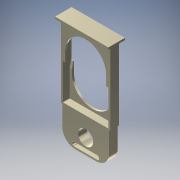
# Autodesk Inventor part: Cup_Dispenser_Slider
Saved by Autodesk Inventor 2016 (Build 200138000, 138)
## iProperties
Created: 2015-07-03
Part Number: Cup_Dispenser_Slider
Material: Generic
Document SubType Name: Modeling
Designer: bastli
Density: 1 g/cm^3
Appearance: Nickel
Author: bastli
Autodesk Inventor part; units mm, degrees
ref_plane "YZ Plane" through (0, 0, 0) normal (1, 0, 0) x (0, 1, 0)
ref_plane "XZ Plane" through (0, 0, 0) normal (0, 1, 0) x (-1, 0, 0)
ref_plane "XY Plane" through (0, 0, 0) normal (0, 0, 1) x (1, 0, 0)
sketch "Sketch13" plane through (0, 0, 0) normal (0, 1, 0) x (-1, 0, 0)
  circle A0 centre (0, 0) radius 35 construction
  circle A1 centre (0, 0) radius 31.375 construction
  line L0 (0, 60.7625) -> (0, -56.1294) construction
  line L1 (45.182, 0) -> (-48.0239, 0) construction
  circle A2 centre (0, 35) radius 35 construction
  circle A3 centre (0, 35) radius 31.375 construction
  line L2 (31.375, 35) -> (31.375, 19.4884)
  line L3 (35, 19.4884) -> (35, 70)
  line L4 (35, 70) -> (0, 70)
  line L5 (31.375, 19.4884) -> (35, 19.4884)
  arc A4 (31.375, 35) -> (0, 66.375) centre (0, 35) ccw
  line L6 (0, 70) -> (0, 66.375) construction
  line L7 (0, 31.375) -> (0, 3.625) construction
  line L8 (0, 17.5) -> (45.182, 17.5) construction
  line L9 (-31.375, 35) -> (-31.375, 19.4884)
  line L10 (-35, 19.4884) -> (-35, 70)
  line L11 (-35, 70) -> (0, 70)
  line L12 (-31.375, 19.4884) -> (-35, 19.4884)
  arc A5 (0, 66.375) -> (-31.375, 35) centre (0, 35) ccw
  line L13 (31.375, 0) -> (31.375, 15.5116)
  line L14 (35, 15.5116) -> (35, -35)
  line L15 (35, -35) -> (0, -35)
  line L16 (31.375, 15.5116) -> (35, 15.5116)
  arc A6 (0, -31.375) -> (31.375, 0) centre (0, 0) ccw
  line L17 (-35, 15.5116) -> (-35, -35)
  line L18 (-35, -35) -> (0, -35)
  line L19 (-31.375, 15.5116) -> (-35, 15.5116)
  line L20 (-31.375, 0) -> (-31.375, 15.5116)
  arc A7 (-31.375, 0) -> (0, -31.375) centre (0, 0) ccw
  line L21 (35, 70) -> (35, -35)
  line L22 (-35, -35) -> (-35, 70)
  line L23 (-38, 73) -> (38, 73)
  line L24 (38, 73) -> (38, -38)
  line L25 (38, -38) -> (-38, -38)
  line L26 (-38, -38) -> (-38, 73)
  line L27 (-38, 73) -> (38, -38) construction
  line L28 (38, 73) -> (-38, -38) construction
  dimension "d49" = 70
  dimension "d50" = 62.75
  dimension "d51" = 70
  dimension "d53" = 62.75
  dimension "d54" = 76
  dimension "d55" = 111
  constraints: 58 end point, 15 symmetric about line, 13 point on circle, 6 centre point, 6 point on line, 4 coincident, 4 parallel, 4 perpendicular, 3 horizontal, 3 midpoint, 3 tangent, 2 vertical alignment, 1 collinear, 1 vertical, 7 other
  measures "d51" diameter of A2
  measures "d53" diameter of A3
  measures "d54" distance of L24.end L25.end
  measures "d55" distance of L23.end L24.end
extrude "Extrusion11" add sketch "Sketch13" against normal blind 3 contours L14 L15 L18 L17 L19 L20 A7 A6 L13 L16 | L23 L24 L25 L26
extrude "Extrusion12" add sketch "Sketch13" against normal blind 10.5
sketch "Sketch14" plane through (0, -10.5, 0) normal (0, -1, 0) x (1, 0, 0)
  arc A0 (31.375, 35) -> (0, 66.375) centre (0, 35) ccw projected
  line L0 (31.375, 35) -> (31.375, 19.4884) projected
  line L1 (31.375, 19.4884) -> (35, 19.4884) projected
  arc A1 (0, 66.375) -> (-31.375, 35) centre (0, 35) ccw projected
  line L2 (-31.375, 35) -> (-31.375, 19.4884) projected
  line L3 (-31.375, 19.4884) -> (-35, 19.4884) projected
  line L4 (-35, 70) -> (35, 70) projected
  line L5 (35, 70) -> (35, -35) projected
  line L6 (-35, -35) -> (-35, 70) projected
  line L7 (35, 70) -> (35, -35) projected
  line L8 (35, -35) -> (-35, -35) projected
  line L9 (-35, -35) -> (-35, 70) projected
  line L10 (-35, 70) -> (35, 70) projected
  line L11 (38, 73) -> (-38, 73) projected
  line L12 (-38, 73) -> (-38, -38) projected
  line L13 (-38, -38) -> (38, -38) projected
  line L14 (38, -38) -> (38, 73) projected
  point P0 (0, 0)
extrude "Extrusion13" add sketch "Sketch14" along normal blind 3 contours A0 A1 L2 L3 L6 L4 L5 L1 L0 | L14 L13 L12 L11
chamfer "Chamfer3" distance 2 angle 45 2 edges at (-38, -6.75, -38) (38, -6.75, -38)
chamfer "Chamfer4" distance 10 distance2 2 1 edges at (33.1875, -3, 15.5116) measured on face at (33.1875, -3, 15.0116)
chamfer "Chamfer5" distance 10 distance2 2 1 edges at (-33.1875, -3, 15.5116) measured on face at (-33.1875, -3, 15.0116)
chamfer "Chamfer6" distance 2 distance2 10 1 edges at (-33.1875, -10.5, 19.4884) measured on face at (-33.1875, -11, 19.4884)
chamfer "Chamfer7" distance 2 distance2 10 1 edges at (33.1875, -10.5, 19.4884) measured on face at (33.1875, -11, 19.4884)
sketch "Sketch18" plane through (-35, 0, 70) normal (1, 0, 0) x (0, 0, -1)
  line L0 (38, -10.5) -> (35, -7.5)
  line L1 (35, -7.5) -> (32, -10.5)
  line L2 (40.5116, -10.5) -> (0, -10.5) projected
  line L3 (35, -10.5) -> (35, -13.5) construction
  line L4 (35, -10.5) -> (35, -7.5) construction
  point P0 (70, 0)
  dimension "d85" = 45
  dimension "d86" = 3
  constraints: 6 end point, 3 point on line, 1 perpendicular, 1 vertical
  measures "d85" angle of L2 L0
  measures "d86" distance from line of L2 L0.end
extrude "Extrusion17" add sketch "Sketch18" along normal up to surface (3.625 mm away)
mirror "Mirror4" about plane through (0, 0, 0) normal (1, 0, 0) of "Extrusion17"
sketch "Sketch15" plane through (-38, 0, 73) normal (0, 0, 1) x (1, 0, 0)
  line L0 (76, 0) -> (0, 0) projected
  line L1 (0, 0) -> (0, -13.5) projected
  line L2 (76, -13.5) -> (0, -13.5) projected
  line L3 (76, 0) -> (76, -13.5) projected
  point P0 (38, 0)
extrude "Extrusion14" add sketch "Sketch15" along normal blind 3
sketch "Sketch16" plane through (-38, 0, 76) normal (0, 0, 1) x (1, 0, 0)
  line L0 (76, 0) -> (0, 0) projected
  line L1 (0, 0) -> (0, -13.5) projected
  line L2 (0, -13.5) -> (76, -13.5) projected
  line L3 (76, -13.5) -> (76, 0) projected
  line L4 (76, 0) -> (76, -13.5) projected
  line L5 (76, -13.5) -> (0, -13.5) projected
  line L6 (0, -13.5) -> (0, 0) projected
  line L7 (0, 0) -> (76, 0) projected
  line L8 (-3, -19.5) -> (79, -19.5) projected
  line L9 (79, -19.5) -> (79, 6) projected
  line L10 (-3, 6) -> (79, 6) projected
  line L11 (-3, -19.5) -> (-3, 6) projected
  point P0 (38, 0)
extrude "Extrusion15" add sketch "Sketch16" along normal blind 3 contours L3 L2 L1 L0 | L11 L10 L9 L8
sketch "Sketch21" plane through (36, -13.5, -38) normal (0, 0, -1) x (-1, 0, 0)
  line L0 (0, 0) -> (0, 13.5) projected
  line L1 (72, 0) -> (0, 0) projected
  line L2 (72, 13.5) -> (72, 0) projected
  line L3 (72, 13.5) -> (0, 13.5) projected
  point P0 (36, 13.5)
extrude "Extrusion20" add sketch "Sketch21" along normal blind 50
sketch "Sketch22" plane through (0, -13.5, 0) normal (0, -1, 0) x (1, 0, 0)
  line L0 (36, -88) -> (-36, -88) projected
  line L1 (0, -88) -> (0, -22.6471) construction
  line L2 (-17.5, -82) -> (17.5, -82) construction
  line L3 (-17.5, -85) -> (17.5, -85)
  line L4 (17.5, -79) -> (-17.5, -79)
  arc A0 (-17.5, -79) -> (-17.5, -85) centre (-17.5, -82) ccw
  arc A1 (17.5, -85) -> (17.5, -79) centre (17.5, -82) ccw
  line L5 (-36, -38) -> (-36, -88) projected
  line L6 (36, -38) -> (36, -88) projected
  line L7 (-16, -88) -> (16, -88)
  line L8 (36, -68) -> (36, -38)
  line L9 (-38, -36) -> (-36, -38) projected
  line L10 (-36, -38) -> (-36, -68)
  arc A2 (16, -88) -> (36, -68) centre (16, -68) ccw
  arc A3 (-36, -68) -> (-16, -88) centre (-16, -68) ccw
  line L11 (-36, -68) -> (-36, -88)
  line L12 (-36, -88) -> (-16, -88)
  line L13 (-36, -88) -> (36, -88) projected
  line L14 (16, -88) -> (36, -88)
  line L15 (36, -88) -> (36, -68)
  circle A4 centre (0, -64.5) radius 11.5 projected
  point P0 (0, 0)
  point P1 (0, -82)
  dimension "d97" = 35
  dimension "d98" = 3
  dimension "d99" = 3
  dimension "d100" = 20
  constraints: 24 end point, 12 tangent, 8 point on circle, 6 point on line, 5 collinear, 4 centre point, 2 midpoint, 2 perpendicular, 1 equal radius, 1 parallel, 1 vertical
  measures "d97" distance of L2.end L2.start
  measures "d98" distance between parallel lines of L3 L2
  measures "d99" distance between parallel lines of L3 L0
  measures "d100" radius of A2
extrude "Extrusion21" cut sketch "Sketch22" against normal up to surface (13.5 mm away)
chamfer "Chamfer8" distance 1 angle 45 4 edges at (20.5, 0, -82) (0, 0, -79) (-20.5, 0, -82) (0, 0, -85)
thicken "Thicken1" operation add thickness 0.1 both sides no extend neighbours yes toward (0, 0, 1) faces at (12.6667, -17.5, 76) (-0.4621, -13.5, -41.0279) (-27.3942, 0, -55.0519) (-38, -9, 38.6667) (38, -9, 1.3333) (36, -4.5, -58) (32.5248, -4.5, -79.2664) (5.3333, -4.5, -88) (5.8333, -9.3333, -79) (-17.9812, -5.1667, -79.0388) (-33.3205, -4.5, -78) (20.4976, -5.1667, -81.8792) (-5.8333, -9.3333, -85) (-36, -9, -58) (-37.3333, -4.5, -36.6667) (37.3333, -9, -36.6667)
equation "\"printer_offset\" = 0.2"
body "Solid2"
